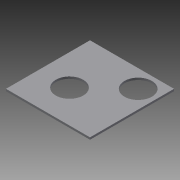
# Autodesk Inventor part: Element
Saved by Autodesk Inventor 2015 (Build 190159000, 159)
## iProperties
Created: 2016-03-23
Part Number: Element
Material: Generic
Document SubType Name: Modeling
Designer: Noah
Density: 1 g/cm^3
Appearance: Default
Author: Noah
Autodesk Inventor part; units mm, degrees
ref_plane "YZ Plane" through (0, 0, 0) normal (1, 0, 0) x (0, 1, 0)
ref_plane "XZ Plane" through (0, 0, 0) normal (0, 1, 0) x (-1, 0, 0)
ref_plane "XY Plane" through (0, 0, 0) normal (0, 0, 1) x (1, 0, 0)
sketch "Sketch1" plane through (0, 0, 0) normal (0, 0, 1) x (1, 0, 0)
  line L0 (-164, 164) -> (164, 164)
  line L1 (164, 164) -> (164, -164)
  line L2 (164, -164) -> (-164, -164)
  line L3 (-164, -164) -> (-164, 164)
  point P0 (0, 0)
  dimension "d0" = 328
  dimension "d1" = 328
  dimension "d2" = 164
  dimension "d3" = 164
  constraints: 8 end point, 2 parallel, 1 horizontal, 1 perpendicular
  measures "d0" distance of L0.start L0.end
  measures "d1" distance of L2.end L0.start
  measures "d2" distance from line of point (0, 0) L1
  measures "d3" distance from line of point (0, 0) L0
extrude "Extrusion1" add sketch "Sketch1" along normal blind 8
sketch "Sketch3" plane through (0, 0, 0) normal (0, 0, -1) x (-1, 0, 0)
  circle A0 centre (-94, 94) radius 53.5
  circle A1 centre (44, -36) radius 53.5
  circle A2 centre (44, -36) radius 12.5 construction
  circle A3 centre (-94, 94) radius 12.5 construction
  point P0 (0, 0)
  dimension "d18" = 107
  dimension "d19" = 107
  constraints: 2 centre point, 2 concentric
  measures "d18" diameter of A1
  measures "d19" diameter of A0
extrude "Extrusion2" cut sketch "Sketch3" against normal through all
sketch "Sketch4" plane through (0, 0, 0) normal (0, 0, -1) x (-1, 0, 0)
  line L0 (110.61, 53.21) -> (110.61, -98.79) projected
  line L1 (111.61, -99.79) -> (159.35, -99.79) projected
  line L2 (160.35, -98.79) -> (160.35, 53.21) projected
  line L3 (159.35, 54.21) -> (111.61, 54.21) projected
  line L4 (154, 61.21) -> (55.35, 61.21) projected
  line L5 (55.35, 98.21) -> (154, 98.21) projected
  line L6 (55.35, 61.21) -> (55.35, 98.21) projected
  line L7 (155.35, 61.21) -> (155.35, 98.21) projected
  arc A0 (110.61, -98.79) -> (111.61, -99.79) centre (111.61, -98.79) ccw projected
  arc A1 (159.35, -99.79) -> (160.35, -98.79) centre (159.35, -98.79) ccw projected
  arc A2 (160.35, 53.21) -> (159.35, 54.21) centre (159.35, 53.21) ccw projected
  arc A3 (111.61, 54.21) -> (110.61, 53.21) centre (111.61, 53.21) ccw projected
  line L8 (154, 61.21) -> (155.35, 61.21) projected
  line L9 (155.35, 98.21) -> (154, 98.21) projected
  point P0 (0, 0)
extrude "Extrusion3" cut sketch "Sketch4" against normal through all
sketch "Sketch5" plane through (0, 0, 0) normal (0, 0, -1) x (-1, 0, 0)
  line L0 (-79, -7) -> (-79, -155) construction
  line L1 (-163, -7) -> (-79, -7) construction
  line L2 (-163, -155) -> (-163, -7) construction
  line L3 (-79, -155) -> (-163, -155) construction
  line L4 (-83, -146) -> (-83, -16)
  line L5 (-88, -11) -> (-154, -11)
  line L6 (-159, -16) -> (-159, -146)
  line L7 (-154, -151) -> (-88, -151)
  arc A0 (-88, -151) -> (-83, -146) centre (-88, -146) ccw
  arc A1 (-159, -146) -> (-154, -151) centre (-154, -146) ccw
  arc A2 (-154, -11) -> (-159, -16) centre (-154, -16) ccw
  arc A3 (-83, -16) -> (-88, -11) centre (-88, -16) ccw
  point P0 (0, 0)
  dimension "d20" = 4
  dimension "d21" = 5
  constraints: 8 end point, 8 point on circle, 8 tangent, 4 centre point, 3 equal radius, 3 other
  measures "d20" distance between parallel lines of L0 L4
  measures "d21" radius of A0
extrude "Extrusion4" cut sketch "Sketch5" against normal through all
equation "\"d0\" = edge_length - 2 * wall_width"
equation "\"d1\" = edge_length - 2 * wall_width"
equation "\"d2\" = -wall_width + 0.5 * edge_length"
equation "\"d3\" = -wall_width + 0.5 * edge_length"
equation "\"d4\" = wall_width_small"
equation "\"edge_length\" = 360"
equation "\"wall_width\" = 16"
equation "\"wall_width_small\" = 8"
body "Solid1"
